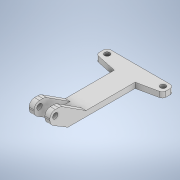
# Autodesk Inventor part: camera_mount
Saved by Autodesk Inventor 2020 (Build 240168000, 168)
## iProperties
Created: 2023-05-24
Part Number: camera_mount
Material: Типовые
Document SubType Name: Modeling
Designer: Администратор
Density: 1 g/cm^3
Appearance: По умолчанию
Author: Администратор
Autodesk Inventor part; units mm, degrees
ref_plane "YZ Plane" through (0, 0, 0) normal (1, 0, 0) x (0, 1, 0)
ref_plane "XZ Plane" through (0, 0, 0) normal (0, 1, 0) x (-1, 0, 0)
ref_plane "XY Plane" through (0, 0, 0) normal (0, 0, 1) x (1, 0, 0)
sketch "Эскиз1" plane through (0, 0, 0) normal (0, 1, 0) x (-1, 0, 0)
  line L0 (18.5, 23) -> (-18.5, 23) construction
  line L1 (-18.5, -18.6138) -> (-18.5, -21) construction
  line L2 (-16.5, -23) -> (16.5, -23) construction
  line L3 (18.5, -21) -> (18.5, 23) construction
  line L4 (18.5, 23) -> (-18.5, -23) construction
  line L5 (-18.5, 23) -> (18.5, -23) construction
  line L6 (18.5, -21) -> (18.5, -18.6138) construction
  line L7 (18.5, -13) -> (-18.5, -13) construction
  circle A0 centre (15.5, -20) radius 1.5 construction
  line L8 (18.5, -23) -> (18.5, -18.6138) construction
  line L9 (0, 23) -> (0, -23) construction
  circle A1 centre (-15.5, -20) radius 1.5 construction
  line L10 (0, -13) -> (16.9227, -16.659) construction
  line L11 (0, -13) -> (-16.9227, -16.659) construction
  arc A2 (18.5, -18.6138) -> (16.9227, -16.659) centre (16.5, -18.6138) ccw construction
  arc A3 (16.5, -23) -> (18.5, -21) centre (16.5, -21) ccw construction
  arc A4 (-16.9227, -16.659) -> (-18.5, -18.6138) centre (-16.5, -18.6138) ccw construction
  arc A5 (-18.5, -21) -> (-16.5, -23) centre (-16.5, -21) ccw construction
  line L12 (-18.5, -18.6138) -> (-18.5, -21) construction
  line L13 (0, 23) -> (5.75, 23) construction
  line L14 (5.75, 23) -> (-5.75, 23) construction
  line L15 (-5.75, 23) -> (-5.75, -14.2432) construction
  line L16 (5.75, 23) -> (5.75, -14.2432) construction
  line L17 (-5.75, 23) -> (5.75, 23)
  line L18 (5.75, 23) -> (5.75, -14.2432)
  line L19 (5.75, -14.2432) -> (16.9227, -16.659)
  line L20 (16.5, -23) -> (-16.5, -23)
  line L21 (-16.9227, -16.659) -> (-5.75, -14.2432)
  line L22 (-5.75, -14.2432) -> (-5.75, 23)
  arc A6 (18.5, -18.6138) -> (16.9227, -16.659) centre (16.5, -18.6138) ccw
  arc A7 (16.5, -23) -> (18.5, -21) centre (16.5, -21) ccw
  line L23 (18.5, -18.6138) -> (18.5, -21)
  arc A8 (-16.9227, -16.659) -> (-18.5, -18.6138) centre (-16.5, -18.6138) ccw
  arc A9 (-18.5, -21) -> (-16.5, -23) centre (-16.5, -21) ccw
  line L24 (-18.5, -18.6138) -> (-18.5, -21)
  circle A10 centre (15.5, -20) radius 1.5
  circle A11 centre (-15.5, -20) radius 1.5
  point P0 (0, 0)
  dimension "d0" = 37
  dimension "d1" = 46
  dimension "d2" = 10
  dimension "d3" = 3
  dimension "d4" = 3
  dimension "d5" = 3
  dimension "d8" = 2
  dimension "d9" = 5.75
  dimension "d10" = 11.5
  dimension "d11" = 2
  dimension "d12" = 2
  constraints: 50 end point, 18 point on line, 16 point on circle, 16 tangent, 12 centre point, 7 equal radius, 5 midpoint, 5 perpendicular, 4 collinear, 3 parallel, 2 coincident, 2 horizontal, 2 vertical, 1 symmetric about line, 1 other
  measures "d0" distance of L5.end L4.end
  measures "d1" distance of L4.end L0.end
  measures "d2" distance of L5.end L7.start
  measures "d3" diameter of A0
  measures "d4" distance from line of L2 A0.centre
  measures "d5" distance from line of L3 A0.centre
  measures "d8" radius of A2
  measures "d9" distance of L9.start L13.end
  measures "d10" distance of L13.end L14.end
  measures "d11" radius of A6
  measures "d12" radius of A8
extrude "Выдавливание1" add sketch "Эскиз1" along normal blind 3
sketch "Эскиз2" plane through (0, 0, 0) normal (1, 0, 0) x (0, 1, 0)
  line L0 (0, 23) -> (6, 23) construction
  line L1 (8.2648, 33) -> (12, 33) construction
  line L2 (12, 30) -> (12, 28.1748)
  line L3 (12, 13) -> (0, 13) construction
  line L4 (0, 13) -> (0, 33) construction
  line L5 (0, 33) -> (12, 13) construction
  line L6 (12, 33) -> (0, 13) construction
  circle A0 centre (9, 30) radius 1.5 construction
  line L7 (12, 33) -> (12, 27) construction
  line L8 (11.3647, 26.0118) -> (3, 13)
  line L9 (3, 23) -> (3, -14.2432) construction
  line L10 (9, 33) -> (6, 33) construction
  line L11 (4.8348, 31.058) -> (0, 23)
  arc A1 (12, 30) -> (9, 33) centre (9, 30) ccw
  arc A2 (11.3647, 26.0118) -> (12, 28.1748) centre (8, 28.1748) ccw
  arc A3 (8.2648, 33) -> (4.8348, 31.058) centre (8.2648, 29) ccw
  line L12 (8.2648, 33) -> (9, 33)
  circle A4 centre (9, 30) radius 1.5
  line L13 (0, -14.2432) -> (0, 23) projected
  line L14 (3, -14.2432) -> (3, 23) projected
  line L15 (0, 23) -> (3, 23)
  line L16 (3, 23) -> (3, 13)
  point P0 (0, 0)
  dimension "d15" = 6
  dimension "d16" = 12
  dimension "d17" = 20
  dimension "d18" = 3
  dimension "d19" = 3
  dimension "d20" = 3
  dimension "d21" = 6
  dimension "d22" = 6
  dimension "d23" = 3
  dimension "d24" = 4
  constraints: 28 end point, 10 point on line, 6 point on circle, 6 tangent, 5 centre point, 3 horizontal, 2 equal radius, 2 midpoint, 2 parallel, 2 perpendicular, 1 coincident, 1 collinear
  measures "d15" distance of L0.start L0.end
  measures "d16" distance of L3.start L3.end
  measures "d17" distance of L1.end L3.start
  measures "d18" diameter of A0
  measures "d19" distance from line of L1 A0.centre
  measures "d20" distance from line of L2 A0.centre
  measures "d21" distance of L1.end L7.end
  measures "d22" distance of L1.end L10.end
  measures "d23" radius of A1
  measures "d24" radius of A2
extrude "Выдавливание2" add sketch "Эскиз2" along normal mid plane 11.5
extrude "Выдавливание3" cut sketch "Эскиз2" along normal mid plane 6
